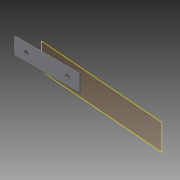
# Autodesk Inventor part: Hopper Bracing P12 to P1
Saved by Autodesk Inventor 2014 SP1 (Build 180222100, 222)
## iProperties
Created: 2013-12-18
Part Number: Hopper Bracing P12 to P1
Material: Aluminum 6061
Document SubType Name: Modeling
Designer: Moses
Mass: 1.35366 g
Surface Area: 13.7526 cm^2
Volume: 0.499505 cm^3
Density: 2.71 g/cm^3
Appearance: Aluminum - Flat
Author: Moses
Autodesk Inventor part; units mm, degrees
ref_plane "YZ Plane" through (0, 0, 0) normal (1, 0, 0) x (0, 1, 0)
ref_plane "XZ Plane" through (0, 0, 0) normal (0, 1, 0) x (-1, 0, 0)
sketch "Sketch1" plane through (0, 0, 0) normal (0, 0, 1) x (1, 0, 0)
  line L0 (0, 0) -> (50.8, 0)
  line L1 (50.8, 0) -> (50.8, 12.7)
  line L2 (50.8, 12.7) -> (0, 12.7)
  line L3 (0, 12.7) -> (0, 0)
  line L4 (25.4, 12.7) -> (25.4, 0) construction
  line L5 (9.525, 6.35) -> (41.275, 6.35) construction
  circle A0 centre (9.525, 6.35) radius 1.5875
  circle A1 centre (41.275, 6.35) radius 1.5875
  point P0 (25.4, 6.35)
  dimension "d0" = 12.7
  dimension "d1" = 50.8
  dimension "d2" = 3.175
  dimension "d3" = 9.525
  constraints: 12 end point, 4 midpoint, 2 centre point, 2 coincident, 2 horizontal, 2 parallel, 1 equal radius, 1 perpendicular
  measures "d0" distance of L0.end L1.end
  measures "d1" distance of L0.start L0.end
  measures "d2" diameter of A0
  measures "d3" distance from line of L5.start L3
extrude "Extrusion1" add sketch "Sketch1" along normal blind 0.7937 contours L3 L2 L1 L0 | A1
ref_plane "Work Plane2" through (117.4846, -2.3812, 5.6317) normal (-0.0842, 0, 0.9965) x (0, 1, 0)
sketch "Sketch2" plane through (117.4846, -2.3812, 5.6317) normal (-0.0842, 0, 0.9965) x (0, 1, 0)
  circle A0 centre (8.7312, 76.2) radius 1.5875 projected
  line L0 (18.2562, 0) -> (0, 0) construction
  line L1 (18.2562, 0) -> (18.2562, 92.075) construction
  line L2 (0, 92.075) -> (18.2562, 92.075) construction
  line L3 (0, 0) -> (0, 92.075) construction
  point P0 (2.3812, 117.5418)
extrude "Extrusion2" cut sketch "Sketch2" along normal through all
body "Solid1"
